Autodesk Inventor part; units mm, degrees
(part 3 of 4)
  measures "d35" distance of L140.end L141.end
  measures "d36" distance of L147.end L148.end
  measures "d37" distance of L146.end L147.end
  measures "d38" distance of L153.end L154.end
  measures "d39" distance of L152.end L153.end
  measures "d40" distance of L159.end L160.end
  measures "d41" distance of L158.end L159.end
  measures "d42" distance of L165.end L166.end
  measures "d43" distance of L164.end L165.end
  measures "d44" distance of L171.end L172.end
  measures "d45" distance of L170.end L171.end
  measures "d46" distance of L177.end L178.end
  measures "d47" distance of L176.end L177.end
  measures "d48" distance of L183.end L184.end
  measures "d49" distance of L182.end L183.end
  measures "d50" distance of L189.end L190.end
  measures "d51" distance of L188.end L189.end
  measures "d52" distance of L195.end L196.end
  measures "d53" distance of L194.end L195.end
  measures "d54" distance of L201.end L202.end
  measures "d55" distance of L200.end L201.end
  measures "d56" distance of L207.end L208.end
  measures "d57" distance of L206.end L207.end
  measures "d58" distance of L213.end L214.end
  measures "d59" distance of L212.end L213.end
  measures "d60" distance of L219.end L220.end
  measures "d61" distance of L218.end L219.end
  measures "d62" distance of L225.end L226.end
  measures "d63" distance of L224.end L225.end
  measures "d64" distance of L231.end L232.end
extrude "Thin plate" add sketch "Sketch1" along normal blind 0.25 contours L87 L101 L102 L103 L98 A100 L291 L290 L293 L292 L97 L96 L95 L93 L92 L91 L86 L85 L84 L83 L82 L81 L80 L79 L88 L77
sketch "Sketch3" plane through (0, 0, 0.25) normal (0, 0, 1) x (1, 0, 0)
  line L0 (222.1338, -62.3704) -> (222.1338, -26.6088) projected
  arc A0 (218.9918, -21.6745) -> (222.1338, -26.6088) centre (220, -24.5) ccw projected
  line L1 (218.9918, -21.6745) -> (206.7063, -21.6745) projected
  line L2 (206.7063, -21.6745) -> (206.7063, -7.6695) projected
  line L3 (206.7063, -7.6695) -> (220.7113, -7.6695) projected
  line L4 (220.7113, -7.6695) -> (220.7113, -21.5855) projected
  arc A1 (222.1338, -22.3912) -> (220.7113, -21.5855) centre (220, -24.5) ccw projected
  line L5 (222.1338, -22.3912) -> (222.1338, 32.8296) projected
  line L6 (222.1338, 32.8296) -> (51.6148, 32.8296) projected
  line L7 (51.6148, 32.8296) -> (51.6148, 61.3884) projected
  line L8 (51.6148, 61.3884) -> (4.6528, 61.3884) projected
  line L9 (4.6528, 61.3884) -> (4.6528, 37.758) projected
  line L10 (4.6528, 37.758) -> (14.4318, 37.758) projected
  line L11 (14.4318, 37.758) -> (14.4318, 13.7046) projected
  line L12 (14.4318, 13.7046) -> (4.6528, 13.7046) projected
  line L13 (4.6528, 13.7046) -> (4.6528, -5.1455) projected
  line L14 (4.6528, -5.1455) -> (9.8598, -5.1455) projected
  line L15 (9.8598, -5.1455) -> (9.8598, -24.3954) projected
  line L16 (9.8598, -24.3954) -> (0.2048, -24.3954) projected
  line L17 (0.2048, -24.3954) -> (0.2048, -49.0614) projected
  line L18 (0.2048, -49.0614) -> (8.6302, -49.0614) projected
  line L19 (8.6302, -49.0614) -> (8.6302, -62.3704) projected
  line L20 (8.6302, -62.3704) -> (57.4568, -62.3704) projected
  line L21 (57.4568, -62.3704) -> (57.4568, -43.3204) projected
  line L22 (57.4568, -43.3204) -> (148.1338, -43.3204) projected
  line L23 (148.1338, -43.3204) -> (148.1338, -62.3704) projected
  line L24 (148.1338, -62.3704) -> (222.1338, -62.3704) projected
  line L25 (206.7063, -52.274) -> (219.1063, -52.274) projected
  line L26 (219.1063, -52.274) -> (219.1063, -58.274) projected
  line L27 (219.1063, -58.274) -> (206.7063, -58.274) projected
  line L28 (206.7063, -58.274) -> (206.7063, -52.274) projected
  line L29 (206.7063, -34.274) -> (206.7063, -28.274) projected
  line L30 (206.7063, -28.274) -> (219.1063, -28.274) projected
  line L31 (219.1063, -28.274) -> (219.1063, -34.274) projected
  line L32 (219.1063, -34.274) -> (206.7063, -34.274) projected
  line L33 (175.2108, -45.7695) -> (181.2108, -45.7695) projected
  line L34 (181.2108, -45.7695) -> (181.2108, -58.1695) projected
  line L35 (181.2108, -58.1695) -> (175.2108, -58.1695) projected
  line L36 (175.2108, -58.1695) -> (175.2108, -45.7695) projected
  line L37 (151.2108, -58.1695) -> (151.2108, -45.7695) projected
  line L38 (151.2108, -45.7695) -> (157.2108, -45.7695) projected
  line L39 (157.2108, -45.7695) -> (157.2108, -58.1695) projected
  line L40 (157.2108, -58.1695) -> (151.2108, -58.1695) projected
  line L41 (52.6683, -14.3724) -> (65.0683, -14.3724) projected
  line L42 (65.0683, -14.3724) -> (65.0683, -20.3724) projected
  line L43 (65.0683, -20.3724) -> (52.6683, -20.3724) projected
  line L44 (52.6683, -20.3724) -> (52.6683, -14.3724) projected
  line L45 (52.6683, 9.6276) -> (65.0683, 9.6276) projected
  line L46 (65.0683, 9.6276) -> (65.0683, 3.6276) projected
  line L47 (65.0683, 3.6276) -> (52.6683, 3.6276) projected
  line L48 (52.6683, 3.6276) -> (52.6683, 9.6276) projected
  line L49 (54.4468, -26.8179) -> (60.4468, -26.8179) projected
  line L50 (60.4468, -26.8179) -> (60.4468, -39.2179) projected
  line L51 (60.4468, -39.2179) -> (54.4468, -39.2179) projected
  line L52 (54.4468, -39.2179) -> (54.4468, -26.8179) projected
  line L53 (30.4468, -26.8179) -> (36.4468, -26.8179) projected
  line L54 (36.4468, -26.8179) -> (36.4468, -39.2179) projected
  line L55 (36.4468, -39.2179) -> (30.4468, -39.2179) projected
  line L56 (30.4468, -39.2179) -> (30.4468, -26.8179) projected
  line L57 (159.2083, -45.7695) -> (173.2133, -45.7695) projected
  line L58 (173.2133, -45.7695) -> (173.2133, -59.7745) projected
  line L59 (173.2133, -59.7745) -> (159.2083, -59.7745) projected
  line L60 (159.2083, -59.7745) -> (159.2083, -45.7695) projected
  line L61 (187.6563, -45.7695) -> (201.6613, -45.7695) projected
  line L62 (201.6613, -45.7695) -> (201.6613, -59.7745) projected
  line L63 (201.6613, -59.7745) -> (187.6563, -59.7745) projected
  line L64 (187.6563, -59.7745) -> (187.6563, -45.7695) projected
  line L65 (206.7063, -36.2715) -> (220.7113, -36.2715) projected
  line L66 (220.7113, -36.2715) -> (220.7113, -50.2765) projected
  line L67 (220.7113, -50.2765) -> (206.7063, -50.2765) projected
  line L68 (206.7063, -50.2765) -> (206.7063, -36.2715) projected
  line L69 (201.6613, -26.7195) -> (201.6613, -40.7245) projected
  line L70 (201.6613, -40.7245) -> (187.6563, -40.7245) projected
  line L71 (187.6563, -40.7245) -> (187.6563, -26.7195) projected
  line L72 (187.6563, -26.7195) -> (201.6613, -26.7195) projected
  line L73 (182.6113, -40.7245) -> (168.6063, -40.7245) projected
  line L74 (168.6063, -40.7245) -> (168.6063, -26.7195) projected
  line L75 (168.6063, -26.7195) -> (182.6113, -26.7195) projected
  line L76 (182.6113, -26.7195) -> (182.6113, -40.7245) projected
  line L77 (163.5613, -26.7195) -> (163.5613, -40.7245) projected
  line L78 (163.5613, -40.7245) -> (149.5563, -40.7245) projected
  line L79 (149.5563, -40.7245) -> (149.5563, -26.7195) projected
  line L80 (149.5563, -26.7195) -> (163.5613, -26.7195) projected
  line L81 (187.6563, -7.6695) -> (201.6613, -7.6695) projected
  line L82 (201.6613, -7.6695) -> (201.6613, -21.6745) projected
  line L83 (201.6613, -21.6745) -> (187.6563, -21.6745) projected
  line L84 (187.6563, -21.6745) -> (187.6563, -7.6695) projected
  line L85 (168.6063, -7.6695) -> (182.6113, -7.6695) projected
  line L86 (182.6113, -7.6695) -> (182.6113, -21.6745) projected
  line L87 (182.6113, -21.6745) -> (168.6063, -21.6745) projected
  line L88 (168.6063, -21.6745) -> (168.6063, -7.6695) projected
  line L89 (149.5563, -7.6695) -> (163.5613, -7.6695) projected
  line L90 (163.5613, -7.6695) -> (163.5613, -21.6745) projected
  line L91 (163.5613, -21.6745) -> (149.5563, -21.6745) projected
  line L92 (149.5563, -21.6745) -> (149.5563, -7.6695) projected
  line L93 (220.7113, 11.3805) -> (220.7113, -2.6245) projected
  line L94 (220.7113, -2.6245) -> (206.7063, -2.6245) projected
  line L95 (206.7063, -2.6245) -> (206.7063, 11.3805) projected
  line L96 (206.7063, 11.3805) -> (220.7113, 11.3805) projected
  line L97 (187.6563, 11.3805) -> (201.6613, 11.3805) projected
  line L98 (201.6613, 11.3805) -> (201.6613, -2.6245) projected
  line L99 (201.6613, -2.6245) -> (187.6563, -2.6245) projected
  line L100 (187.6563, -2.6245) -> (187.6563, 11.3805) projected
  line L101 (168.6063, 11.3805) -> (182.6113, 11.3805) projected
  line L102 (182.6113, 11.3805) -> (182.6113, -2.6245) projected
  line L103 (182.6113, -2.6245) -> (168.6063, -2.6245) projected
  line L104 (168.6063, -2.6245) -> (168.6063, 11.3805) projected
  line L105 (149.5563, 11.3805) -> (163.5613, 11.3805) projected
  line L106 (163.5613, 11.3805) -> (163.5613, -2.6245) projected
  line L107 (163.5613, -2.6245) -> (149.5563, -2.6245) projected
  line L108 (149.5563, -2.6245) -> (149.5563, 11.3805) projected
  line L109 (220.7113, 30.4305) -> (220.7113, 16.4255) projected
  line L110 (220.7113, 16.4255) -> (206.7063, 16.4255) projected
  line L111 (206.7063, 16.4255) -> (206.7063, 30.4305) projected
  line L112 (206.7063, 30.4305) -> (220.7113, 30.4305) projected
  line L113 (187.6563, 30.4305) -> (201.6613, 30.4305) projected
  line L114 (201.6613, 30.4305) -> (201.6613, 16.4255) projected
  line L115 (201.6613, 16.4255) -> (187.6563, 16.4255) projected
  line L116 (187.6563, 16.4255) -> (187.6563, 30.4305) projected
  line L117 (168.6063, 30.4305) -> (182.6113, 30.4305) projected
  line L118 (182.6113, 30.4305) -> (182.6113, 16.4255) projected
  line L119 (182.6113, 16.4255) -> (168.6063, 16.4255) projected
  line L120 (168.6063, 16.4255) -> (168.6063, 30.4305) projected
  line L121 (149.5563, 30.4305) -> (163.5613, 30.4305) projected
  line L122 (163.5613, 30.4305) -> (163.5613, 16.4255) projected
  line L123 (163.5613, 16.4255) -> (149.5563, 16.4255) projected
  line L124 (149.5563, 16.4255) -> (149.5563, 30.4305) projected
  line L125 (87.5555, 30.3969) -> (101.5605, 30.3969) projected
  line L126 (101.5605, 30.3969) -> (101.5605, 16.3919) projected
  line L127 (101.5605, 16.3919) -> (87.5555, 16.3919) projected
  line L128 (87.5555, 16.3919) -> (87.5555, 30.3969) projected
  line L129 (116.1515, 30.3969) -> (130.1565, 30.3969) projected
  line L130 (130.1565, 30.3969) -> (130.1565, 16.3919) projected
  line L131 (130.1565, 16.3919) -> (116.1515, 16.3919) projected
  line L132 (116.1515, 16.3919) -> (116.1515, 30.3969) projected
  line L133 (120.9275, -26.7671) -> (134.9325, -26.7671) projected
  line L134 (134.9325, -26.7671) -> (134.9325, -40.7721) projected
  line L135 (134.9325, -40.7721) -> (120.9275, -40.7721) projected
  line L136 (120.9275, -40.7721) -> (120.9275, -26.7671) projected
  line L137 (101.8775, -7.7171) -> (115.8825, -7.7171) projected
  line L138 (115.8825, -7.7171) -> (115.8825, -21.7221) projected
  line L139 (115.8825, -21.7221) -> (101.8775, -21.7221) projected
  line L140 (101.8775, -21.7221) -> (101.8775, -7.7171) projected
  line L141 (101.8775, -26.7671) -> (115.8825, -26.7671) projected
  line L142 (115.8825, -26.7671) -> (115.8825, -40.7721) projected
  line L143 (115.8825, -40.7721) -> (101.8775, -40.7721) projected
  line L144 (101.8775, -40.7721) -> (101.8775, -26.7671) projected
  line L145 (82.8275, -26.7671) -> (96.8325, -26.7671) projected
  line L146 (96.8325, -26.7671) -> (96.8325, -40.7721) projected
  line L147 (96.8325, -40.7721) -> (82.8275, -40.7721) projected
  line L148 (82.8275, -40.7721) -> (82.8275, -26.7671) projected
  line L149 (37.9363, -45.8679) -> (51.9413, -45.8679) projected
  line L150 (51.9413, -45.8679) -> (51.9413, -59.8729) projected
  line L151 (51.9413, -59.8729) -> (37.9363, -59.8729) projected
  line L152 (37.9363, -59.8729) -> (37.9363, -45.8679) projected
  line L153 (14.0603, -45.8679) -> (28.0653, -45.8679) projected
  line L154 (28.0653, -45.8679) -> (28.0653, -59.8729) projected
  line L155 (28.0653, -59.8729) -> (14.0603, -59.8729) projected
  line L156 (14.0603, -59.8729) -> (14.0603, -45.8679) projected
  line L157 (38.4443, -26.8179) -> (52.4493, -26.8179) projected
  line L158 (52.4493, -26.8179) -> (52.4493, -40.8229) projected
  line L159 (52.4493, -40.8229) -> (38.4443, -40.8229) projected
  line L160 (38.4443, -40.8229) -> (38.4443, -26.8179) projected
  line L161 (2.6303, -26.8179) -> (16.6353, -26.8179) projected
  line L162 (16.6353, -26.8179) -> (16.6353, -40.8229) projected
  line L163 (16.6353, -40.8229) -> (2.6303, -40.8229) projected
  line L164 (2.6303, -40.8229) -> (2.6303, -26.8179) projected
  line L165 (52.6683, 1.6301) -> (66.6733, 1.6301) projected
  line L166 (66.6733, 1.6301) -> (66.6733, -12.3749) projected
  line L167 (66.6733, -12.3749) -> (52.6683, -12.3749) projected
  line L168 (52.6683, -12.3749) -> (52.6683, 1.6301) projected
  line L169 (31.3323, -7.7679) -> (45.3373, -7.7679) projected
  line L170 (45.3373, -7.7679) -> (45.3373, -21.7729) projected
  line L171 (45.3373, -21.7729) -> (31.3323, -21.7729) projected
  line L172 (31.3323, -21.7729) -> (31.3323, -7.7679) projected
  line L173 (12.2823, -7.7679) -> (26.2873, -7.7679) projected
  line L174 (26.2873, -7.7679) -> (26.2873, -21.7729) projected
  line L175 (26.2873, -21.7729) -> (12.2823, -21.7729) projected
  line L176 (12.2823, -21.7729) -> (12.2823, -7.7679) projected
  line L177 (26.2523, 11.2821) -> (40.2573, 11.2821) projected
  line L178 (40.2573, 11.2821) -> (40.2573, -2.7229) projected
  line L179 (40.2573, -2.7229) -> (26.2523, -2.7229) projected
  line L180 (26.2523, -2.7229) -> (26.2523, 11.2821) projected
  line L181 (7.2023, 11.2821) -> (21.2073, 11.2821) projected
  line L182 (21.2073, 11.2821) -> (21.2073, -2.7229) projected
  line L183 (21.2073, -2.7229) -> (7.2023, -2.7229) projected
  line L184 (7.2023, -2.7229) -> (7.2023, 11.2821) projected
  line L185 (54.9543, 30.3321) -> (68.9593, 30.3321) projected
  line L186 (68.9593, 30.3321) -> (68.9593, 16.3271) projected
  line L187 (68.9593, 16.3271) -> (54.9543, 16.3271) projected
  line L188 (54.9543, 16.3271) -> (54.9543, 30.3321) projected
  line L189 (35.9043, 30.3321) -> (49.9093, 30.3321) projected
  line L190 (49.9093, 30.3321) -> (49.9093, 16.3271) projected
  line L191 (49.9093, 16.3271) -> (35.9043, 16.3271) projected
  line L192 (35.9043, 16.3271) -> (35.9043, 30.3321) projected
  line L193 (16.8543, 30.3321) -> (30.8593, 30.3321) projected
  line L194 (30.8593, 30.3321) -> (30.8593, 16.3271) projected
  line L195 (30.8593, 16.3271) -> (16.8543, 16.3271) projected
  line L196 (16.8543, 16.3271) -> (16.8543, 30.3321) projected
  line L197 (33.3643, 58.9889) -> (47.3693, 58.9889) projected
  line L198 (47.3693, 58.9889) -> (47.3693, 44.9839) projected
  line L199 (47.3693, 44.9839) -> (33.3643, 44.9839) projected
  line L200 (33.3643, 44.9839) -> (33.3643, 58.9889) projected
  line L201 (9.4883, 58.9889) -> (23.4933, 58.9889) projected
  line L202 (23.4933, 58.9889) -> (23.4933, 44.9839) projected
  line L203 (23.4933, 44.9839) -> (9.4883, 44.9839) projected
  line L204 (9.4883, 44.9839) -> (9.4883, 58.9889) projected
  line L205 (148.1338, -62.3704) -> (148.1338, 32.8296) projected
  line L206 (137.43, -43.2696) -> (137.43, -24.2696) projected
  line L207 (137.43, -24.2696) -> (118.38, -24.2696) projected
  line L208 (118.38, -24.2696) -> (118.38, -5.2196) projected
  line L209 (118.38, -5.2196) -> (99.38, -5.2196) projected
  line L210 (99.38, -5.2196) -> (99.38, -24.2696) projected
  line L211 (99.38, -24.2696) -> (80.33, -24.2696) projected
  line L212 (80.33, -24.2696) -> (80.33, -43.2696) projected
  line L213 (80.33, 13.8944) -> (80.33, 32.8296) projected
  line L214 (137.43, 13.8944) -> (80.33, 13.8944) projected
  line L215 (137.43, 32.8296) -> (137.43, 13.8944) projected
  line L216 (71.4568, -43.3204) -> (71.4568, 32.8296) projected
  line L217 (51.6148, 42.3884) -> (-66.3852, 42.3884) projected
  line L218 (71.4568, 32.8296) -> (-223.6412, 32.8296) projected
  line L219 (80.33, -43.2696) -> (137.43, -43.2696)
  line L220 (57.4568, -43.3204) -> (148.1338, -43.3204) projected
  point P0 (0, 0)
  point P1 (4.6528, 42.3884)
  point P2 (14.4318, 32.8296)
  constraints: 2 end point, 1 parallel
extrude "Switch supports" add sketch "Sketch3" along normal blind 3 contours L24 L23 L205 L6 L5 A1 L4 L3 L2 L1 A0 L0 | L22 L21 L20 L19 L18 L17 L16 L15 L14 L13 L12 L11 L218 L6 L216 | L215 L214 L213 L6 | L217 L9 L8 L7 | L219 L212 L211 L210 L209 L208 L207 L206
sketch "Sketch4" plane through (0, 0, 0) normal (0, 0, -1) x (-1, 0, 0)
  line L0 (-222.1338, -62.3704) -> (-222.1338, -26.6088) construction
  line L1 (-148.1338, -62.3704) -> (-222.1338, -62.3704) construction
  line L2 (-148.1338, -43.3204) -> (-148.1338, -62.3704) construction
  line L3 (-57.4568, -43.3204) -> (-148.1338, -43.3204) construction
  line L4 (-57.4568, -62.3704) -> (-57.4568, -43.3204) construction
  line L5 (-8.6302, -62.3704) -> (-57.4568, -62.3704) construction
  line L6 (-8.6302, -49.0614) -> (-8.6302, -62.3704) construction
  line L7 (-0.2048, -49.0614) -> (-8.6302, -49.0614) construction
  line L8 (-0.2048, -24.3954) -> (-0.2048, -49.0614) construction
  line L9 (-9.8598, -24.3954) -> (-0.2048, -24.3954) construction
  line L10 (-9.8598, -5.1455) -> (-9.8598, -24.3954) construction
  line L11 (-4.6528, -5.1455) -> (-9.8598, -5.1455) construction
  line L12 (-4.6528, 13.7046) -> (-4.6528, -5.1455) construction
  line L13 (-14.4318, 13.7046) -> (-4.6528, 13.7046) construction
  line L14 (-14.4318, 37.758) -> (-14.4318, 13.7046) construction
  line L15 (-4.6528, 37.758) -> (-14.4318, 37.758) construction
  line L16 (-4.6528, 61.3884) -> (-4.6528, 37.758) construction
  line L17 (-51.6148, 61.3884) -> (-4.6528, 61.3884) construction
  line L18 (-51.6148, 32.8296) -> (-51.6148, 61.3884) construction
  line L19 (-222.1338, 32.8296) -> (-51.6148, 32.8296) construction
  line L20 (-222.1338, -22.3912) -> (-222.1338, 32.8296) construction
  arc A0 (-220.7113, -21.5855) -> (-222.1338, -22.3912) centre (-220, -24.5) ccw construction
  line L21 (-220.7113, -7.6695) -> (-220.7113, -21.5855) construction
  line L22 (-206.7063, -7.6695) -> (-220.7113, -7.6695) construction
  line L23 (-206.7063, -21.6745) -> (-206.7063, -7.6695) construction
  line L24 (-218.9918, -21.6745) -> (-206.7063, -21.6745) construction
  arc A1 (-222.1338, -26.6088) -> (-218.9918, -21.6745) centre (-220, -24.5) ccw construction
  line L25 (-206.7063, -52.274) -> (-219.1063, -52.274) construction
  line L26 (-206.7063, -58.274) -> (-206.7063, -52.274) construction
  line L27 (-219.1063, -58.274) -> (-206.7063, -58.274) construction
  line L28 (-219.1063, -52.274) -> (-219.1063, -58.274) construction
  line L29 (-206.7063, -34.274) -> (-206.7063, -28.274) construction
  line L30 (-219.1063, -34.274) -> (-206.7063, -34.274) construction
  line L31 (-219.1063, -28.274) -> (-219.1063, -34.274) construction
  line L32 (-206.7063, -28.274) -> (-219.1063, -28.274) construction
  line L33 (-175.2108, -45.7695) -> (-181.2108, -45.7695) construction
  line L34 (-175.2108, -58.1695) -> (-175.2108, -45.7695) construction
  line L35 (-181.2108, -58.1695) -> (-175.2108, -58.1695) construction
  line L36 (-181.2108, -45.7695) -> (-181.2108, -58.1695) construction
  line L37 (-151.2108, -58.1695) -> (-151.2108, -45.7695) construction
  line L38 (-157.2108, -58.1695) -> (-151.2108, -58.1695) construction
  line L39 (-157.2108, -45.7695) -> (-157.2108, -58.1695) construction
  line L40 (-151.2108, -45.7695) -> (-157.2108, -45.7695) construction
  line L41 (-52.6683, -14.3724) -> (-65.0683, -14.3724) construction
  line L42 (-52.6683, -20.3724) -> (-52.6683, -14.3724) construction
  line L43 (-65.0683, -20.3724) -> (-52.6683, -20.3724) construction
  line L44 (-65.0683, -14.3724) -> (-65.0683, -20.3724) construction
  line L45 (-52.6683, 9.6276) -> (-65.0683, 9.6276) construction
  line L46 (-52.6683, 3.6276) -> (-52.6683, 9.6276) construction
  line L47 (-65.0683, 3.6276) -> (-52.6683, 3.6276) construction
  line L48 (-65.0683, 9.6276) -> (-65.0683, 3.6276) construction
  line L49 (-54.4468, -26.8179) -> (-60.4468, -26.8179) construction
  line L50 (-54.4468, -39.2179) -> (-54.4468, -26.8179) construction
  line L51 (-60.4468, -39.2179) -> (-54.4468, -39.2179) construction
  line L52 (-60.4468, -26.8179) -> (-60.4468, -39.2179) construction
  line L53 (-30.4468, -26.8179) -> (-36.4468, -26.8179) construction
  line L54 (-30.4468, -39.2179) -> (-30.4468, -26.8179) construction
  line L55 (-36.4468, -39.2179) -> (-30.4468, -39.2179) construction
  line L56 (-36.4468, -26.8179) -> (-36.4468, -39.2179) construction
  line L57 (-159.2083, -45.7695) -> (-173.2133, -45.7695) construction
  line L58 (-159.2083, -59.7745) -> (-159.2083, -45.7695) construction
  line L59 (-173.2133, -59.7745) -> (-159.2083, -59.7745) construction
  line L60 (-173.2133, -45.7695) -> (-173.2133, -59.7745) construction
  line L61 (-187.6563, -45.7695) -> (-201.6613, -45.7695) construction
  line L62 (-187.6563, -59.7745) -> (-187.6563, -45.7695) construction
  line L63 (-201.6613, -59.7745) -> (-187.6563, -59.7745) construction
  line L64 (-201.6613, -45.7695) -> (-201.6613, -59.7745) construction
  line L65 (-206.7063, -36.2715) -> (-220.7113, -36.2715) construction
  line L66 (-206.7063, -50.2765) -> (-206.7063, -36.2715) construction
  line L67 (-220.7113, -50.2765) -> (-206.7063, -50.2765) construction
  line L68 (-220.7113, -36.2715) -> (-220.7113, -50.2765) construction
  line L69 (-201.6613, -26.7195) -> (-201.6613, -40.7245) construction
  line L70 (-187.6563, -26.7195) -> (-201.6613, -26.7195) construction
  line L71 (-187.6563, -40.7245) -> (-187.6563, -26.7195) construction
  line L72 (-201.6613, -40.7245) -> (-187.6563, -40.7245) construction
  line L73 (-182.6113, -40.7245) -> (-168.6063, -40.7245) construction
  line L74 (-182.6113, -26.7195) -> (-182.6113, -40.7245) construction
  line L75 (-168.6063, -26.7195) -> (-182.6113, -26.7195) construction
  line L76 (-168.6063, -40.7245) -> (-168.6063, -26.7195) construction
  line L77 (-163.5613, -26.7195) -> (-163.5613, -40.7245) construction
  line L78 (-149.5563, -26.7195) -> (-163.5613, -26.7195) construction
  line L79 (-149.5563, -40.7245) -> (-149.5563, -26.7195) construction
  line L80 (-163.5613, -40.7245) -> (-149.5563, -40.7245) construction
  line L81 (-187.6563, -7.6695) -> (-201.6613, -7.6695) construction
  line L82 (-187.6563, -21.6745) -> (-187.6563, -7.6695) construction
  line L83 (-201.6613, -21.6745) -> (-187.6563, -21.6745) construction
  line L84 (-201.6613, -7.6695) -> (-201.6613, -21.6745) construction
  line L85 (-168.6063, -7.6695) -> (-182.6113, -7.6695) construction
  line L86 (-168.6063, -21.6745) -> (-168.6063, -7.6695) construction
  line L87 (-182.6113, -21.6745) -> (-168.6063, -21.6745) construction
  line L88 (-182.6113, -7.6695) -> (-182.6113, -21.6745) construction
  line L89 (-149.5563, -7.6695) -> (-163.5613, -7.6695) construction
  line L90 (-149.5563, -21.6745) -> (-149.5563, -7.6695) construction
  line L91 (-163.5613, -21.6745) -> (-149.5563, -21.6745) construction
  line L92 (-163.5613, -7.6695) -> (-163.5613, -21.6745) construction
  line L93 (-220.7113, 11.3805) -> (-220.7113, -2.6245) construction
  line L94 (-206.7063, 11.3805) -> (-220.7113, 11.3805) construction
  line L95 (-206.7063, -2.6245) -> (-206.7063, 11.3805) construction
  line L96 (-220.7113, -2.6245) -> (-206.7063, -2.6245) construction
  line L97 (-187.6563, 11.3805) -> (-201.6613, 11.3805) construction
  line L98 (-187.6563, -2.6245) -> (-187.6563, 11.3805) construction
  line L99 (-201.6613, -2.6245) -> (-187.6563, -2.6245) construction
  line L100 (-201.6613, 11.3805) -> (-201.6613, -2.6245) construction
  line L101 (-168.6063, 11.3805) -> (-182.6113, 11.3805) construction
  line L102 (-168.6063, -2.6245) -> (-168.6063, 11.3805) construction
  line L103 (-182.6113, -2.6245) -> (-168.6063, -2.6245) construction
  line L104 (-182.6113, 11.3805) -> (-182.6113, -2.6245) construction
  line L105 (-149.5563, 11.3805) -> (-163.5613, 11.3805) construction
  line L106 (-149.5563, -2.6245) -> (-149.5563, 11.3805) construction
  line L107 (-163.5613, -2.6245) -> (-149.5563, -2.6245) construction
  line L108 (-163.5613, 11.3805) -> (-163.5613, -2.6245) construction
  line L109 (-220.7113, 30.4305) -> (-220.7113, 16.4255) construction
  line L110 (-206.7063, 30.4305) -> (-220.7113, 30.4305) construction
  line L111 (-206.7063, 16.4255) -> (-206.7063, 30.4305) construction
  line L112 (-220.7113, 16.4255) -> (-206.7063, 16.4255) construction
  line L113 (-187.6563, 30.4305) -> (-201.6613, 30.4305) construction
  line L114 (-187.6563, 16.4255) -> (-187.6563, 30.4305) construction
  line L115 (-201.6613, 16.4255) -> (-187.6563, 16.4255) construction
  line L116 (-201.6613, 30.4305) -> (-201.6613, 16.4255) construction
  line L117 (-168.6063, 30.4305) -> (-182.6113, 30.4305) construction
  line L118 (-168.6063, 16.4255) -> (-168.6063, 30.4305) construction
  line L119 (-182.6113, 16.4255) -> (-168.6063, 16.4255) construction
  line L120 (-182.6113, 30.4305) -> (-182.6113, 16.4255) construction
  line L121 (-149.5563, 30.4305) -> (-163.5613, 30.4305) construction
  line L122 (-149.5563, 16.4255) -> (-149.5563, 30.4305) construction
  line L123 (-163.5613, 16.4255) -> (-149.5563, 16.4255) construction
  line L124 (-163.5613, 30.4305) -> (-163.5613, 16.4255) construction
  line L125 (-87.5555, 30.3969) -> (-101.5605, 30.3969) construction
  line L126 (-87.5555, 16.3919) -> (-87.5555, 30.3969) construction
  line L127 (-101.5605, 16.3919) -> (-87.5555, 16.3919) construction
  line L128 (-101.5605, 30.3969) -> (-101.5605, 16.3919) construction
  line L129 (-116.1515, 30.3969) -> (-130.1565, 30.3969) construction
  line L130 (-116.1515, 16.3919) -> (-116.1515, 30.3969) construction
  line L131 (-130.1565, 16.3919) -> (-116.1515, 16.3919) construction
  line L132 (-130.1565, 30.3969) -> (-130.1565, 16.3919) construction
  line L133 (-120.9275, -26.7671) -> (-134.9325, -26.7671) construction
  line L134 (-120.9275, -40.7721) -> (-120.9275, -26.7671) construction
  line L135 (-134.9325, -40.7721) -> (-120.9275, -40.7721) construction
  line L136 (-134.9325, -26.7671) -> (-134.9325, -40.7721) construction
  line L137 (-101.8775, -7.7171) -> (-115.8825, -7.7171) construction
  line L138 (-101.8775, -21.7221) -> (-101.8775, -7.7171) construction
  line L139 (-115.8825, -21.7221) -> (-101.8775, -21.7221) construction
  line L140 (-115.8825, -7.7171) -> (-115.8825, -21.7221) construction
  line L141 (-101.8775, -26.7671) -> (-115.8825, -26.7671) construction
  line L142 (-101.8775, -40.7721) -> (-101.8775, -26.7671) construction
  line L143 (-115.8825, -40.7721) -> (-101.8775, -40.7721) construction
  line L144 (-115.8825, -26.7671) -> (-115.8825, -40.7721) construction
  line L145 (-82.8275, -26.7671) -> (-96.8325, -26.7671) construction
  line L146 (-82.8275, -40.7721) -> (-82.8275, -26.7671) construction
  line L147 (-96.8325, -40.7721) -> (-82.8275, -40.7721) construction
  line L148 (-96.8325, -26.7671) -> (-96.8325, -40.7721) construction
  line L149 (-37.9363, -45.8679) -> (-51.9413, -45.8679) construction
  line L150 (-37.9363, -59.8729) -> (-37.9363, -45.8679) construction
  line L151 (-51.9413, -59.8729) -> (-37.9363, -59.8729) construction
  line L152 (-51.9413, -45.8679) -> (-51.9413, -59.8729) construction
  line L153 (-14.0603, -45.8679) -> (-28.0653, -45.8679) construction
  line L154 (-14.0603, -59.8729) -> (-14.0603, -45.8679) construction
  line L155 (-28.0653, -59.8729) -> (-14.0603, -59.8729) construction
  line L156 (-28.0653, -45.8679) -> (-28.0653, -59.8729) construction
  line L157 (-38.4443, -26.8179) -> (-52.4493, -26.8179) construction
  line L158 (-38.4443, -40.8229) -> (-38.4443, -26.8179) construction
  line L159 (-52.4493, -40.8229) -> (-38.4443, -40.8229) construction
  line L160 (-52.4493, -26.8179) -> (-52.4493, -40.8229) construction
  line L161 (-2.6303, -26.8179) -> (-16.6353, -26.8179) construction
  line L162 (-2.6303, -40.8229) -> (-2.6303, -26.8179) construction
  line L163 (-16.6353, -40.8229) -> (-2.6303, -40.8229) construction
  line L164 (-16.6353, -26.8179) -> (-16.6353, -40.8229) construction
  line L165 (-52.6683, 1.6301) -> (-66.6733, 1.6301) construction
  line L166 (-52.6683, -12.3749) -> (-52.6683, 1.6301) construction
  line L167 (-66.6733, -12.3749) -> (-52.6683, -12.3749) construction
  line L168 (-66.6733, 1.6301) -> (-66.6733, -12.3749) construction
  line L169 (-31.3323, -7.7679) -> (-45.3373, -7.7679) construction
  line L170 (-31.3323, -21.7729) -> (-31.3323, -7.7679) construction
  line L171 (-45.3373, -21.7729) -> (-31.3323, -21.7729) construction
  line L172 (-45.3373, -7.7679) -> (-45.3373, -21.7729) construction
  line L173 (-12.2823, -7.7679) -> (-26.2873, -7.7679) construction
  line L174 (-12.2823, -21.7729) -> (-12.2823, -7.7679) construction
  line L175 (-26.2873, -21.7729) -> (-12.2823, -21.7729) construction
  line L176 (-26.2873, -7.7679) -> (-26.2873, -21.7729) construction
  line L177 (-26.2523, 11.2821) -> (-40.2573, 11.2821) construction
  line L178 (-26.2523, -2.7229) -> (-26.2523, 11.2821) construction
  line L179 (-40.2573, -2.7229) -> (-26.2523, -2.7229) construction
  line L180 (-40.2573, 11.2821) -> (-40.2573, -2.7229) construction
  line L181 (-7.2023, 11.2821) -> (-21.2073, 11.2821) construction
  line L182 (-7.2023, -2.7229) -> (-7.2023, 11.2821) construction
  line L183 (-21.2073, -2.7229) -> (-7.2023, -2.7229) construction
  line L184 (-21.2073, 11.2821) -> (-21.2073, -2.7229) construction
  line L185 (-54.9543, 30.3321) -> (-68.9593, 30.3321) construction
  line L186 (-54.9543, 16.3271) -> (-54.9543, 30.3321) construction
  line L187 (-68.9593, 16.3271) -> (-54.9543, 16.3271) construction
  line L188 (-68.9593, 30.3321) -> (-68.9593, 16.3271) construction
  line L189 (-35.9043, 30.3321) -> (-49.9093, 30.3321) construction
  line L190 (-35.9043, 16.3271) -> (-35.9043, 30.3321) construction
  line L191 (-49.9093, 16.3271) -> (-35.9043, 16.3271) construction
  line L192 (-49.9093, 30.3321) -> (-49.9093, 16.3271) construction
  line L193 (-16.8543, 30.3321) -> (-30.8593, 30.3321) construction
  line L194 (-16.8543, 16.3271) -> (-16.8543, 30.3321) construction
  line L195 (-30.8593, 16.3271) -> (-16.8543, 16.3271) construction
  line L196 (-30.8593, 30.3321) -> (-30.8593, 16.3271) construction
  line L197 (-33.3643, 58.9889) -> (-47.3693, 58.9889) construction
  line L198 (-33.3643, 44.9839) -> (-33.3643, 58.9889) construction
  line L199 (-47.3693, 44.9839) -> (-33.3643, 44.9839) construction
  line L200 (-47.3693, 58.9889) -> (-47.3693, 44.9839) construction
  line L201 (-9.4883, 58.9889) -> (-23.4933, 58.9889) construction
  line L202 (-9.4883, 44.9839) -> (-9.4883, 58.9889) construction
  line L203 (-23.4933, 44.9839) -> (-9.4883, 44.9839) construction
  line L204 (-23.4933, 58.9889) -> (-23.4933, 44.9839) construction
  line L205 (-36.4468, -23.3179) -> (-30.4468, -23.3179)
  line L206 (-30.4468, -23.3179) -> (-30.4468, -41.2179)
  line L207 (-30.4468, -41.2179) -> (-36.4468, -41.2179)
  line L208 (-36.4468, -41.2179) -> (-36.4468, -29.3179)
  line L209 (-60.4468, -23.3179) -> (-54.4468, -23.3179)
  line L210 (-54.4468, -29.3179) -> (-54.4468, -41.2179)
  line L211 (-54.4468, -41.2179) -> (-60.4468, -41.2179)
  line L212 (-60.4468, -41.2179) -> (-60.4468, -23.3179)
  line L213 (-67.0683, -14.3724) -> (-67.0683, -20.3724)
  line L214 (-67.0683, -20.3724) -> (-49.1683, -20.3724)
  line L215 (-49.1683, -20.3724) -> (-49.1683, -14.3724)
  line L216 (-49.1683, 9.6276) -> (-67.0683, 9.6276)
  line L217 (-67.0683, 9.6276) -> (-67.0683, 3.6276)
  line L218 (-49.1683, 3.6276) -> (-49.1683, 9.6276)
  line L219 (-181.2108, -42.2695) -> (-175.2108, -42.2695)
  line L220 (-175.2108, -60.1695) -> (-181.2108, -60.1695)
  line L221 (-181.2108, -60.1695) -> (-181.2108, -42.2695)
  line L222 (-157.2108, -42.2695) -> (-151.2108, -42.2695)
  line L223 (-151.2108, -42.2695) -> (-151.2108, -60.1695)
  line L224 (-151.2108, -60.1695) -> (-157.2108, -60.1695)
  line L225 (-157.2108, -60.1695) -> (-157.2108, -48.2695)
  line L226 (-203.2063, -28.274) -> (-221.1063, -28.274)
  line L227 (-221.1063, -28.274) -> (-221.1063, -34.274)
  line L228 (-203.2063, -34.274) -> (-203.2063, -28.274)
  line L229 (-209.2063, -52.274) -> (-221.1063, -52.274)
  line L230 (-221.1063, -52.274) -> (-221.1063, -58.274)
  line L231 (-221.1063, -58.274) -> (-203.2063, -58.274)
  line L232 (-203.2063, -58.274) -> (-203.2063, -52.274)
  line L233 (-206.7063, -28.274) -> (-219.1063, -28.274) projected
  line L234 (-181.2108, -45.7695) -> (-181.2108, -58.1695) projected
  line L235 (-175.2108, -58.1695) -> (-175.2108, -45.7695) projected
  line L236 (-157.2108, -45.7695) -> (-157.2108, -58.1695) projected
  line L237 (-151.2108, -58.1695) -> (-151.2108, -45.7695) projected
  line L238 (-60.4468, -26.8179) -> (-60.4468, -39.2179) projected
  line L239 (-54.4468, -39.2179) -> (-54.4468, -26.8179) projected
  line L240 (-52.6683, -14.3724) -> (-65.0683, -14.3724) projected
  line L241 (-65.0683, 3.6276) -> (-52.6683, 3.6276) projected
  line L242 (-36.4468, -26.8179) -> (-36.4468, -39.2179) projected
  line L243 (-54.4468, -23.3179) -> (-36.4468, -23.3179)
  line L244 (-54.4468, -29.3179) -> (-36.4468, -29.3179)
  line L245 (-49.1683, 3.6276) -> (-49.1683, -14.3724)
  line L246 (-55.1683, 3.6276) -> (-55.1683, -14.3724)
  line L247 (-203.2063, -34.274) -> (-203.2063, -52.274)
  line L248 (-209.2063, -34.274) -> (-209.2063, -52.274)
  line L249 (-175.2108, -42.2695) -> (-157.2108, -42.2695)
  line L250 (-175.2108, -48.2695) -> (-157.2108, -48.2695)
  line L251 (-221.1063, -34.274) -> (-209.2063, -34.274)
  line L252 (-175.2108, -48.2695) -> (-175.2108, -60.1695)
  line L253 (-206.7063, -52.274) -> (-219.1063, -52.274) projected
  line L254 (-67.0683, 3.6276) -> (-55.1683, 3.6276)
  line L255 (-55.1683, -14.3724) -> (-67.0683, -14.3724)
  point P0 (0, 0)
  dimension "d111" = 3.5
  dimension "d112" = 2
  dimension "d113" = 3.5
  dimension "d114" = 2
  dimension "d115" = 3.5
  dimension "d116" = 2
  dimension "d117" = 3.5
  dimension "d118" = 2
  dimension "d119" = 6
  dimension "d120" = 6
  dimension "d121" = 6
  dimension "d122" = 6
  constraints: 84 end point, 17 parallel, 16 collinear, 15 point on line, 13 perpendicular, 9 horizontal, 1 vertical
  measures "d111" distance between parallel lines of L228 L29
  measures "d112" distance between parallel lines of L31 L227
  measures "d113" distance between parallel lines of L33 L219
  measures "d114" distance between parallel lines of L220 L35
  measures "d115" distance between parallel lines of L46 L218
  measures "d116" distance between parallel lines of L217 L48
  measures "d117" distance between parallel lines of L49 L209
  measures "d118" distance between parallel lines of L211 L51
  measures "d119" distance between parallel lines of L247 L248
  measures "d120" distance between parallel lines of L250 L249
  measures "d121" distance between parallel lines of L245 L246
  measures "d122" distance between parallel lines of L244 L243
extrude "Stabilizer cuts" cut sketch "Sketch4" against normal blind 2
sketch "Sketch6" plane through (0, 0, 3.25) normal (0, 0, 1) x (1, 0, 0)
  line L0 (57.4568, -43.3204) -> (71.4568, -43.3204) construction
  line L1 (71.4568, -43.3204) -> (71.4568, 32.8296) construction
  line L2 (71.4568, 32.8296) -> (14.4318, 32.8296) construction
  line L3 (14.4318, 32.8296) -> (14.4318, 13.7046) construction
  line L4 (14.4318, 13.7046) -> (4.6528, 13.7046) construction
  line L5 (4.6528, 13.7046) -> (4.6528, -5.1455) construction
  line L6 (4.6528, -5.1455) -> (9.8598, -5.1455) construction
  line L7 (9.8598, -5.1455) -> (9.8598, -24.3954) construction
  line L8 (9.8598, -24.3954) -> (0.2048, -24.3954) construction
  line L9 (0.2048, -24.3954) -> (0.2048, -49.0614) construction
  line L10 (0.2048, -49.0614) -> (8.6302, -49.0614) construction
  line L11 (8.6302, -49.0614) -> (8.6302, -62.3704) construction
  line L12 (8.6302, -62.3704) -> (57.4568, -62.3704) construction
  line L13 (57.4568, -62.3704) -> (57.4568, -43.3204) construction
  line L14 (16.8543, 30.3321) -> (30.8593, 30.3321) construction
  line L15 (30.8593, 30.3321) -> (30.8593, 16.3271) construction
  line L16 (30.8593, 16.3271) -> (16.8543, 16.3271) construction
  line L17 (16.8543, 16.3271) -> (16.8543, 30.3321) construction
  line L18 (35.9043, 30.3321) -> (49.9093, 30.3321) construction
  line L19 (49.9093, 30.3321) -> (49.9093, 16.3271) construction
  line L20 (49.9093, 16.3271) -> (35.9043, 16.3271) construction
  line L21 (35.9043, 16.3271) -> (35.9043, 30.3321) construction
  line L22 (54.9543, 30.3321) -> (68.9593, 30.3321) construction
  line L23 (68.9593, 30.3321) -> (68.9593, 16.3271) construction
  line L24 (68.9593, 16.3271) -> (54.9543, 16.3271) construction
  line L25 (54.9543, 16.3271) -> (54.9543, 30.3321) construction
  line L26 (7.2023, 11.2821) -> (21.2073, 11.2821) construction
  line L27 (21.2073, 11.2821) -> (21.2073, -2.7229) construction
  line L28 (21.2073, -2.7229) -> (7.2023, -2.7229) construction
  line L29 (7.2023, -2.7229) -> (7.2023, 11.2821) construction
  line L30 (26.2523, 11.2821) -> (40.2573, 11.2821) construction
  line L31 (40.2573, 11.2821) -> (40.2573, -2.7229) construction
  line L32 (40.2573, -2.7229) -> (26.2523, -2.7229) construction
  line L33 (26.2523, -2.7229) -> (26.2523, 11.2821) construction
  line L34 (12.2823, -7.7679) -> (26.2873, -7.7679) construction
  line L35 (26.2873, -7.7679) -> (26.2873, -21.7729) construction
  line L36 (26.2873, -21.7729) -> (12.2823, -21.7729) construction
  line L37 (12.2823, -21.7729) -> (12.2823, -7.7679) construction
  line L38 (31.3323, -7.7679) -> (45.3373, -7.7679) construction
  line L39 (45.3373, -7.7679) -> (45.3373, -21.7729) construction
  line L40 (45.3373, -21.7729) -> (31.3323, -21.7729) construction
  line L41 (31.3323, -21.7729) -> (31.3323, -7.7679) construction
  line L42 (52.6683, 1.6301) -> (66.6733, 1.6301) construction
  line L43 (66.6733, 1.6301) -> (66.6733, -12.3749) construction
  line L44 (66.6733, -12.3749) -> (52.6683, -12.3749) construction
  line L45 (52.6683, -12.3749) -> (52.6683, 1.6301) construction
  line L46 (2.6303, -26.8179) -> (16.6353, -26.8179) construction
  line L47 (16.6353, -26.8179) -> (16.6353, -40.8229) construction
  line L48 (16.6353, -40.8229) -> (2.6303, -40.8229) construction
  line L49 (2.6303, -40.8229) -> (2.6303, -26.8179) construction
  line L50 (38.4443, -26.8179) -> (52.4493, -26.8179) construction
  line L51 (52.4493, -26.8179) -> (52.4493, -40.8229) construction
  line L52 (52.4493, -40.8229) -> (38.4443, -40.8229) construction
  line L53 (38.4443, -40.8229) -> (38.4443, -26.8179) construction
  line L54 (14.0603, -45.8679) -> (28.0653, -45.8679) construction
  line L55 (28.0653, -45.8679) -> (28.0653, -59.8729) construction
  line L56 (28.0653, -59.8729) -> (14.0603, -59.8729) construction
  line L57 (14.0603, -59.8729) -> (14.0603, -45.8679) construction
  line L58 (37.9363, -45.8679) -> (51.9413, -45.8679) construction
  line L59 (51.9413, -45.8679) -> (51.9413, -59.8729) construction
  line L60 (51.9413, -59.8729) -> (37.9363, -59.8729) construction
  line L61 (37.9363, -59.8729) -> (37.9363, -45.8679) construction
  line L62 (30.4468, -26.8179) -> (36.4468, -26.8179) construction
  line L63 (36.4468, -26.8179) -> (36.4468, -39.2179) construction
  line L64 (36.4468, -39.2179) -> (30.4468, -39.2179) construction
  line L65 (30.4468, -39.2179) -> (30.4468, -26.8179) construction
  line L66 (54.4468, -26.8179) -> (60.4468, -26.8179) construction
  line L67 (60.4468, -26.8179) -> (60.4468, -39.2179) construction
  line L68 (60.4468, -39.2179) -> (54.4468, -39.2179) construction
  line L69 (54.4468, -39.2179) -> (54.4468, -26.8179) construction
  line L70 (52.6683, 9.6276) -> (65.0683, 9.6276) construction
  line L71 (65.0683, 9.6276) -> (65.0683, 3.6276) construction
  line L72 (65.0683, 3.6276) -> (52.6683, 3.6276) construction
  line L73 (52.6683, 3.6276) -> (52.6683, 9.6276) construction
  line L74 (52.6683, -14.3724) -> (65.0683, -14.3724) construction
  line L75 (65.0683, -14.3724) -> (65.0683, -20.3724) construction
  line L76 (65.0683, -20.3724) -> (52.6683, -20.3724) construction
  line L77 (52.6683, -20.3724) -> (52.6683, -14.3724) construction
  line L78 (222.1338, 32.8296) -> (148.1338, 32.8296) construction
  line L79 (148.1338, 32.8296) -> (148.1338, -62.3704) construction
  line L80 (148.1338, -62.3704) -> (222.1338, -62.3704) construction
  line L81 (222.1338, -62.3704) -> (222.1338, -26.6088) construction
  arc A0 (218.9918, -21.6745) -> (222.1338, -26.6088) centre (220, -24.5) ccw construction
  line L82 (218.9918, -21.6745) -> (206.7063, -21.6745) construction
  line L83 (206.7063, -21.6745) -> (206.7063, -7.6695) construction
  line L84 (206.7063, -7.6695) -> (220.7113, -7.6695) construction
  line L85 (220.7113, -7.6695) -> (220.7113, -21.5855) construction
  arc A1 (222.1338, -22.3912) -> (220.7113, -21.5855) centre (220, -24.5) ccw construction
  line L86 (222.1338, -22.3912) -> (222.1338, 32.8296) construction
  line L87 (149.5563, 30.4305) -> (163.5613, 30.4305) construction
  line L88 (163.5613, 30.4305) -> (163.5613, 16.4255) construction
  line L89 (163.5613, 16.4255) -> (149.5563, 16.4255) construction
  line L90 (149.5563, 16.4255) -> (149.5563, 30.4305) construction
  line L91 (168.6063, 30.4305) -> (182.6113, 30.4305) construction
  line L92 (182.6113, 30.4305) -> (182.6113, 16.4255) construction
  line L93 (182.6113, 16.4255) -> (168.6063, 16.4255) construction
  line L94 (168.6063, 16.4255) -> (168.6063, 30.4305) construction
  line L95 (187.6563, 30.4305) -> (201.6613, 30.4305) construction
  line L96 (201.6613, 30.4305) -> (201.6613, 16.4255) construction
  line L97 (201.6613, 16.4255) -> (187.6563, 16.4255) construction
  line L98 (187.6563, 16.4255) -> (187.6563, 30.4305) construction
  line L99 (220.7113, 30.4305) -> (220.7113, 16.4255) construction
  line L100 (220.7113, 16.4255) -> (206.7063, 16.4255) construction
  line L101 (206.7063, 16.4255) -> (206.7063, 30.4305) construction
  line L102 (206.7063, 30.4305) -> (220.7113, 30.4305) construction
  line L103 (149.5563, 11.3805) -> (163.5613, 11.3805) construction
  line L104 (163.5613, 11.3805) -> (163.5613, -2.6245) construction
  line L105 (163.5613, -2.6245) -> (149.5563, -2.6245) construction
  line L106 (149.5563, -2.6245) -> (149.5563, 11.3805) construction
  line L107 (168.6063, 11.3805) -> (182.6113, 11.3805) construction
  line L108 (182.6113, 11.3805) -> (182.6113, -2.6245) construction
  line L109 (182.6113, -2.6245) -> (168.6063, -2.6245) construction
  line L110 (168.6063, -2.6245) -> (168.6063, 11.3805) construction
  line L111 (187.6563, 11.3805) -> (201.6613, 11.3805) construction
  line L112 (201.6613, 11.3805) -> (201.6613, -2.6245) construction
  line L113 (201.6613, -2.6245) -> (187.6563, -2.6245) construction
  line L114 (187.6563, -2.6245) -> (187.6563, 11.3805) construction
  line L115 (220.7113, 11.3805) -> (220.7113, -2.6245) construction
  line L116 (220.7113, -2.6245) -> (206.7063, -2.6245) construction
  line L117 (206.7063, -2.6245) -> (206.7063, 11.3805) construction
  line L118 (206.7063, 11.3805) -> (220.7113, 11.3805) construction
  line L119 (149.5563, -7.6695) -> (163.5613, -7.6695) construction
  line L120 (163.5613, -7.6695) -> (163.5613, -21.6745) construction
  line L121 (163.5613, -21.6745) -> (149.5563, -21.6745) construction
  line L122 (149.5563, -21.6745) -> (149.5563, -7.6695) construction
  line L123 (168.6063, -7.6695) -> (182.6113, -7.6695) construction
  line L124 (182.6113, -7.6695) -> (182.6113, -21.6745) construction
  line L125 (182.6113, -21.6745) -> (168.6063, -21.6745) construction
  line L126 (168.6063, -21.6745) -> (168.6063, -7.6695) construction
  line L127 (187.6563, -7.6695) -> (201.6613, -7.6695) construction
  line L128 (201.6613, -7.6695) -> (201.6613, -21.6745) construction
  line L129 (201.6613, -21.6745) -> (187.6563, -21.6745) construction
  line L130 (187.6563, -21.6745) -> (187.6563, -7.6695) construction
  line L131 (163.5613, -26.7195) -> (163.5613, -40.7245) construction
  line L132 (163.5613, -40.7245) -> (149.5563, -40.7245) construction
  line L133 (149.5563, -40.7245) -> (149.5563, -26.7195) construction
  line L134 (149.5563, -26.7195) -> (163.5613, -26.7195) construction
  line L135 (182.6113, -40.7245) -> (168.6063, -40.7245) construction
  line L136 (168.6063, -40.7245) -> (168.6063, -26.7195) construction
  line L137 (168.6063, -26.7195) -> (182.6113, -26.7195) construction
  line L138 (182.6113, -26.7195) -> (182.6113, -40.7245) construction
  line L139 (201.6613, -26.7195) -> (201.6613, -40.7245) construction
  line L140 (201.6613, -40.7245) -> (187.6563, -40.7245) construction
  line L141 (187.6563, -40.7245) -> (187.6563, -26.7195) construction
  line L142 (187.6563, -26.7195) -> (201.6613, -26.7195) construction
  line L143 (206.7063, -36.2715) -> (220.7113, -36.2715) construction
  line L144 (220.7113, -36.2715) -> (220.7113, -50.2765) construction
  line L145 (220.7113, -50.2765) -> (206.7063, -50.2765) construction
  line L146 (206.7063, -50.2765) -> (206.7063, -36.2715) construction
  line L147 (187.6563, -45.7695) -> (201.6613, -45.7695) construction
  line L148 (201.6613, -45.7695) -> (201.6613, -59.7745) construction
  line L149 (201.6613, -59.7745) -> (187.6563, -59.7745) construction
  line L150 (187.6563, -59.7745) -> (187.6563, -45.7695) construction
  line L151 (159.2083, -45.7695) -> (173.2133, -45.7695) construction
  line L152 (173.2133, -45.7695) -> (173.2133, -59.7745) construction
  line L153 (173.2133, -59.7745) -> (159.2083, -59.7745) construction
  line L154 (159.2083, -59.7745) -> (159.2083, -45.7695) construction
  line L155 (151.2108, -58.1695) -> (151.2108, -45.7695) construction
  line L156 (151.2108, -45.7695) -> (157.2108, -45.7695) construction
  line L157 (157.2108, -45.7695) -> (157.2108, -58.1695) construction
  line L158 (157.2108, -58.1695) -> (151.2108, -58.1695) construction
  line L159 (175.2108, -45.7695) -> (181.2108, -45.7695) construction
  line L160 (181.2108, -45.7695) -> (181.2108, -58.1695) construction
  line L161 (181.2108, -58.1695) -> (175.2108, -58.1695) construction
  line L162 (175.2108, -58.1695) -> (175.2108, -45.7695) construction
  line L163 (206.7063, -34.274) -> (206.7063, -28.274) construction
  line L164 (206.7063, -28.274) -> (219.1063, -28.274) construction
  line L165 (219.1063, -28.274) -> (219.1063, -34.274) construction
  line L166 (219.1063, -34.274) -> (206.7063, -34.274) construction
  line L167 (206.7063, -52.274) -> (219.1063, -52.274) construction
  line L168 (219.1063, -52.274) -> (219.1063, -58.274) construction
  line L169 (219.1063, -58.274) -> (206.7063, -58.274) construction
  line L170 (206.7063, -58.274) -> (206.7063, -52.274) construction
  line L171 (32.4468, -26.8179) -> (34.4468, -26.8179)
  line L172 (34.4468, -26.8179) -> (34.4468, -25.8179)
  line L173 (34.4468, -25.8179) -> (32.4468, -25.8179)
  line L174 (32.4468, -25.8179) -> (32.4468, -26.8179)
  line L175 (56.4468, -26.8179) -> (58.4468, -26.8179)
  line L176 (58.4468, -26.8179) -> (58.4468, -25.8179)
  line L177 (58.4468, -25.8179) -> (56.4468, -25.8179)
  line L178 (56.4468, -25.8179) -> (56.4468, -26.8179)
  line L179 (52.6683, 5.6276) -> (51.6683, 5.6276)
  line L180 (51.6683, 5.6276) -> (51.6683, 7.6276)
  line L181 (51.6683, 7.6276) -> (52.6683, 7.6276)
  line L182 (52.6683, 7.6276) -> (52.6683, 5.6276)
  line L183 (52.6683, -18.3724) -> (51.6683, -18.3724)
  line L184 (51.6683, -18.3724) -> (51.6683, -16.3724)
  line L185 (51.6683, -16.3724) -> (52.6683, -16.3724)
  line L186 (52.6683, -16.3724) -> (52.6683, -18.3724)
  line L187 (153.2108, -45.7695) -> (155.2108, -45.7695)
  line L188 (155.2108, -45.7695) -> (155.2108, -44.7695)
  line L189 (155.2108, -44.7695) -> (153.2108, -44.7695)
  line L190 (153.2108, -44.7695) -> (153.2108, -45.7695)
  line L191 (177.2108, -45.7695) -> (179.2108, -45.7695)
  line L192 (179.2108, -45.7695) -> (179.2108, -44.7695)
  line L193 (179.2108, -44.7695) -> (177.2108, -44.7695)
  line L194 (177.2108, -44.7695) -> (177.2108, -45.7695)
  line L195 (206.7063, -58.274) -> (206.7063, -52.274) projected
  line L196 (206.7063, -56.274) -> (205.7063, -56.274)
  line L197 (205.7063, -56.274) -> (205.7063, -54.274)
  line L198 (205.7063, -54.274) -> (206.7063, -54.274)
  line L199 (206.7063, -54.274) -> (206.7063, -56.274)
  line L200 (206.7063, -34.274) -> (206.7063, -28.274) projected
  line L201 (206.7063, -32.274) -> (205.7063, -32.274)
  line L202 (205.7063, -32.274) -> (205.7063, -30.274)
  line L203 (205.7063, -30.274) -> (206.7063, -30.274)
  line L204 (206.7063, -30.274) -> (206.7063, -32.274)
  point P0 (0, 0)
  point P1 (33.4468, -26.8179)
  point P2 (57.4468, -26.8179)
  point P3 (52.6683, 6.6276)
  point P4 (52.6683, -17.3724)
  point P5 (154.2108, -45.7695)
  point P6 (178.2108, -45.7695)
  point P7 (206.7063, -55.274)
  point P8 (206.7063, -31.274)
  dimension "d132" = 2
  dimension "d133" = 1
  dimension "d134" = 2
  dimension "d135" = 1
  dimension "d136" = 1
  dimension "d137" = 2
  dimension "d138" = 1
  dimension "d139" = 2
  dimension "d140" = 2
  dimension "d141" = 1
  dimension "d142" = 2
  dimension "d143" = 1
  dimension "d144" = 1
  dimension "d145" = 2
  dimension "d146" = 1
  dimension "d147" = 2
  constraints: 64 end point, 16 midpoint, 16 parallel, 8 horizontal, 8 perpendicular, 8 point on line
  measures "d132" distance of L173.end L172.end
  measures "d133" distance of L172.end L171.end
  measures "d134" distance of L177.end L176.end
  measures "d135" distance of L176.end L175.end
  measures "d136" distance of L180.end L181.end
  measures "d137" distance of L179.end L180.end
  measures "d138" distance of L184.end L185.end
  measures "d139" distance of L183.end L184.end
  measures "d140" distance of L189.end L188.end
  measures "d141" distance of L188.end L187.end
  measures "d142" distance of L193.end L192.end
  measures "d143" distance of L192.end L191.end
  measures "d144" distance of L197.end L198.end
  measures "d145" distance of L196.end L197.end
  measures "d146" distance of L202.end L203.end
  measures "d147" distance of L201.end L202.end
extrude "Extrusion5" cut sketch "Sketch6" against normal up to surface (3.25 mm away)
sketch "Sketch7" plane through (0, 0, 2) normal (0, 0, -1) x (-1, 0, 0)
  line L0 (-209.2063, -36.2715) -> (-209.2063, -34.274) projected
  line L1 (-203.2063, -28.274) -> (-203.2063, -58.274) projected
  line L2 (-209.2063, -34.274) -> (-203.2063, -34.274)
  line L3 (-203.2063, -34.274) -> (-203.2063, -52.274)
  line L4 (-203.2063, -52.274) -> (-209.2063, -52.274)
  line L5 (-209.2063, -52.274) -> (-209.2063, -34.274)
  line L6 (-206.7063, -52.274) -> (-209.2063, -52.274) projected
  line L7 (-173.2133, -48.2695) -> (-175.2108, -48.2695) projected
  line L8 (-181.2108, -42.2695) -> (-151.2108, -42.2695) projected
  line L9 (-175.2108, -48.2695) -> (-157.2108, -48.2695)
  line L10 (-157.2108, -48.2695) -> (-157.2108, -42.2695)
  line L11 (-157.2108, -42.2695) -> (-175.2108, -42.2695)
  line L12 (-175.2108, -42.2695) -> (-175.2108, -48.2695)
  line L13 (-157.2108, -45.7695) -> (-157.2108, -48.2695) projected
  line L14 (-55.1683, 1.6301) -> (-55.1683, 3.6276) projected
  line L15 (-49.1683, 9.6276) -> (-49.1683, -20.3724) projected
  line L16 (-55.1683, 3.6276) -> (-49.1683, 3.6276)
  line L17 (-49.1683, 3.6276) -> (-49.1683, -14.3724)
  line L18 (-49.1683, -14.3724) -> (-55.1683, -14.3724)
  line L19 (-55.1683, -14.3724) -> (-55.1683, 3.6276)
  line L20 (-52.4493, -29.3179) -> (-54.4468, -29.3179) projected
  line L21 (-60.4468, -23.3179) -> (-30.4468, -23.3179) projected
  line L22 (-54.4468, -29.3179) -> (-36.4468, -29.3179)
  line L23 (-36.4468, -29.3179) -> (-36.4468, -23.3179)
  line L24 (-36.4468, -23.3179) -> (-54.4468, -23.3179)
  line L25 (-54.4468, -23.3179) -> (-54.4468, -29.3179)
  line L26 (-52.6683, -14.3724) -> (-55.1683, -14.3724) projected
  line L27 (-36.4468, -26.8179) -> (-36.4468, -29.3179) projected
  point P0 (0, 0)
  constraints: 32 end point, 8 parallel, 4 collinear, 4 horizontal, 4 perpendicular, 4 point on line
extrude "Extrusion6" cut sketch "Sketch7" against normal blind 0.5
equation "\"d1\" = ipg"
equation "\"d2\" = ipg"
equation "\"d3\" = ipg"